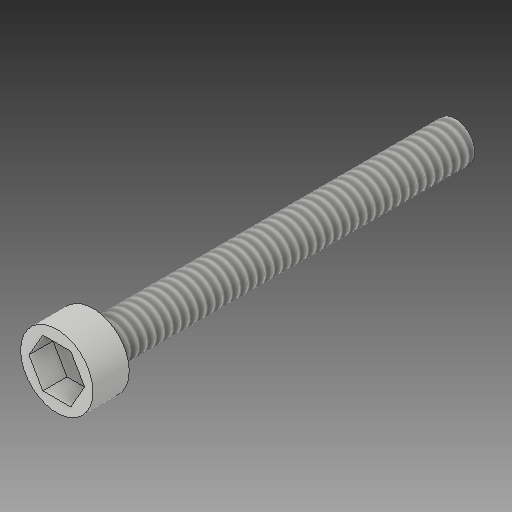
# Autodesk Inventor part: M4 union
Saved by Autodesk Inventor 2019.2 (Build 232265000, 265)
## iProperties
Created: 2018-03-09
Part Number: M4 union
Material: Generic
Document SubType Name: Modeling
Designer: Hogar
Density: 1 g/cm^3
Appearance: Default
Author: Hogar
Autodesk Inventor part; units mm, degrees
ref_plane "YZ Plane" through (0, 0, 0) normal (1, 0, 0) x (0, 1, 0)
ref_plane "XZ Plane" through (0, 0, 0) normal (0, 1, 0) x (-1, 0, 0)
ref_plane "XY Plane" through (0, 0, 0) normal (0, 0, 1) x (1, 0, 0)
sketch "Sketch1" plane through (0, 0, 0) normal (0, 0, 1) x (1, 0, 0)
  circle A0 centre (0, 0) radius 1.621
  dimension "d0" = 3.242
  constraints: 1 centre point, 1 coincident
  measures "d0" diameter of A0
extrude "Extrusion1" add sketch "Sketch1" along normal blind 30
sketch "Sketch2" plane through (0, 0, 30) normal (0, 0, 1) x (1, 0, 0)
  circle A0 centre (0, 0) radius 3
  dimension "d3" = 6
  constraints: 1 centre point, 1 coincident
  measures "d3" diameter of A0
extrude "Extrusion2" add sketch "Sketch2" along normal blind 3
sketch "Sketch3" plane through (0, 0, 33) normal (0, 0, 1) x (1, 0, 0)
  line L0 (1.1547, 2) -> (2.3094, 0)
  line L1 (2.3094, 0) -> (1.1547, -2)
  line L2 (1.1547, -2) -> (-1.1547, -2)
  line L3 (-1.1547, -2) -> (-2.3094, 0)
  line L4 (-2.3094, 0) -> (-1.1547, 2)
  line L5 (-1.1547, 2) -> (1.1547, 2)
  point P0 (0, 0)
  point P1 (0, 0)
  point P2 (0, 2)
  dimension "d7" = 4
  dimension "d9" = 3.4641
  constraints: 12 end point, 1 coincident, 1 midpoint, 13 other
  measures "d7" distance from line of point (0, 2) L2
  measures "d9" horizontal distance of L0.start L3.end
extrude "Extrusion3" cut sketch "Sketch3" against normal blind 2
thread "Thread4" size "M4x0.7" class "6g" standard "ANSI Metric M Profile" full length
body "Solid1"
